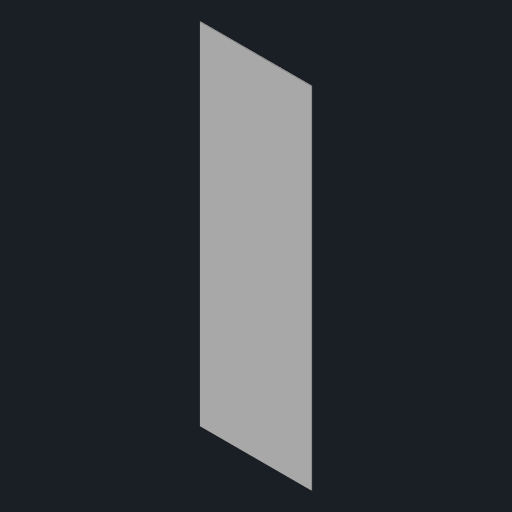
# Autodesk Inventor part: CARCASA_ALUM_7
Saved by Autodesk Inventor 2024.3 (Build 283343000, 343)
## iProperties
Created: 2024-05-15
Part Number: CARCASA_ALUM_7
Material: Generic
Document SubType Name: Sheet Metal
Designer: Niler
Density: 1 g/cm^3
Sheet Metal Rule: Default_mm
Appearance: Default
Author: Niler
Autodesk Inventor part; units mm, degrees
ref_plane "YZ Plane" through (0, 0, 0) normal (1, 0, 0) x (0, 1, 0)
ref_plane "XZ Plane" through (0, 0, 0) normal (0, 1, 0) x (-1, 0, 0)
ref_plane "Work Plane1" through (0, 0, 0) normal (0, 0, 1) x (1, 0, 0)
sketch "Sketch1" plane through (0, 0, 0) normal (0, 0, 1) x (1, 0, 0)
  line L0 (340, -375.7749) -> (340, 375.7749)
  line L1 (100, 375.7749) -> (340, 375.7749)
  line L2 (-102.5, 375.7749) -> (100, 375.7749)
  line L3 (-102.5, 375.7749) -> (-102.5, -375.7749)
  line L4 (100, -375.7749) -> (-102.5, -375.7749)
  line L5 (340, -375.7749) -> (100, -375.7749)
  line L6 (100, 375.7749) -> (100, -375.7749)
  point P0 (0, 0)
extrude "Plate1" add sketch "Sketch1" against normal blind 1.5 contours L5 L6 L1 L0
equation "\"d0\" = Thickness"
equation "\"BendRadius\" = Thickness"
equation "\"BendReliefWidth\" = Thickness"
equation "\"BendReliefDepth\" = 0.5 * Thickness"
equation "\"CornerReliefSize\" = 4 * Thickness"
equation "\"MinimumRemnant\" = 2 * Thickness"
equation "\"TransitionRadius\" = BendRadius"
equation "\"JacobiRadiusSize\" = BendRadius"
equation "\"GapSize\" = Thickness"
equation "\"Thickness\" = 1.5"
body "Solid1"
